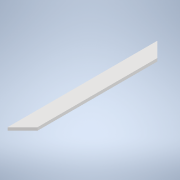
# Autodesk Inventor part: Bridge_width_small
Saved by Autodesk Inventor 2020 (Build 240168000, 168)
## iProperties
Created: 2020-07-03
Part Number: Bridge_width_small
Material: Generic
Document SubType Name: Modeling
Designer: user
Density: 1 g/cm^3
Appearance: Default
Author: user
Autodesk Inventor part; units mm, degrees
ref_plane "YZ Plane" through (0, 0, 0) normal (1, 0, 0) x (0, 1, 0)
ref_plane "XZ Plane" through (0, 0, 0) normal (0, 1, 0) x (-1, 0, 0)
ref_plane "XY Plane" through (0, 0, 0) normal (0, 0, 1) x (1, 0, 0)
sketch "Sketch1" plane through (0, 0, 0) normal (0, 1, 0) x (-1, 0, 0)
  line L0 (13.1128, 53.7694) -> (8.1128, 53.7694)
  line L1 (8.1128, 53.7694) -> (8.1128, 3.7694)
  line L2 (8.1128, 3.7694) -> (13.1128, 3.7694)
  line L3 (13.1128, 3.7694) -> (13.1128, 53.7694)
  line L4 (13.1128, 53.7694) -> (8.1128, 48.7694)
  line L5 (13.1128, 3.7694) -> (8.1128, 8.7694)
  point P0 (0, 0)
  point P1 (-6.8872, 33.7694)
  dimension "d0" = 45
  dimension "d1" = 5
  dimension "d2" = 45
  dimension "d6" = 40
  constraints: 12 end point, 2 parallel, 2 point on line, 1 horizontal, 1 perpendicular
  measures "d0" angle of L4 L0
  measures "d1" distance of L0.end L0.start
  measures "d2" angle of L2 L5
  measures "d6" distance of L5.end L4.end
extrude "Extrusion1" add sketch "Sketch1" along normal blind 1 contours L3 L5 L1 L4
body "Solid1"
